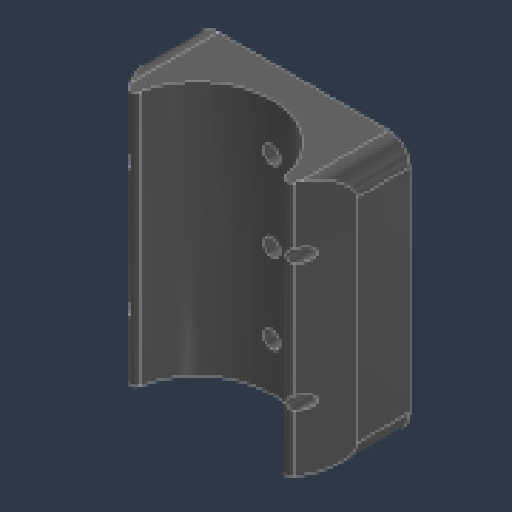
# Autodesk Inventor part: MOUNT,SPARK_MAX,ARM
Saved by Autodesk Inventor 2024.3 (Build 283343000, 343)
## iProperties
Category: _
Manager: _
ILogicPurgeVersion: 0.0.0.0
OnSaveVersion: 2.2.20.20
Created: 2025-03-14
Part Number: MOUNT,SPARK_MAX,ARM
Checked By: 00
Engr Approved By: _
User Status: Work In Process
Material: Nylon 6/6
Description: STANDARD (mm)
Document SubType Name: Modeling
Mfg Approved By: Stephen.Oerton
Designer: John Thibert
Manufacturer: Standard
Standards Organization: Custom
Density: 1.13 g/cm^3
Appearance: Dark Gray
CN_MASS: 0.0
CN_SERVICEABLE: _
FIRST_DESCRIPTION: _
SECOND_DESCRIPTION: _
THIRD_DESCRIPTION: _
ModelCat: Uncategorized
Subject: _
Author: John Thibert
Keywords: -
Revision Number: A
Autodesk Inventor part; units mm, degrees
ref_plane "YZ Plane" through (0, 0, 0) normal (1, 0, 0) x (0, 1, 0)
ref_plane "XZ Plane" through (0, 0, 0) normal (0, 1, 0) x (-1, 0, 0)
ref_plane "XY Plane" through (0, 0, 0) normal (0, 0, 1) x (1, 0, 0)
sketch "Sketch2" plane through (0, 0, 0) normal (0, 0, 1) x (1, 0, 0)
  line L0 (-31.75, -38.1) -> (31.75, -38.1)
  line L1 (31.75, -38.1) -> (31.75, 38.1)
  line L2 (31.75, 38.1) -> (-31.75, 38.1)
  line L3 (-31.75, 38.1) -> (-31.75, -38.1)
  line L4 (-31.75, -38.1) -> (31.75, 38.1) construction
  line L5 (31.75, -38.1) -> (-31.75, 38.1) construction
  point P0 (0, 0)
  dimension "d0" = 63.5
  dimension "d1" = 76.2
  constraints: 12 end point, 2 midpoint, 2 parallel, 1 horizontal, 1 perpendicular
  measures "d0" distance of L2.end L1.end
  measures "d1" distance of L0.end L1.end
extrude "Extrusion1" add sketch "Sketch2" against normal blind 31.75
sketch "Sketch4" plane through (-31.75, 38.1, 0) normal (0, 1, 0) x (1, 0, 0)
  arc A0 (53.975, 0) -> (9.525, 0) centre (31.75, 0) ccw
  line L0 (63.5, 0) -> (0, 0) construction
  line L1 (63.5, 0) -> (63.5, 31.75) projected
  line L2 (0, 31.75) -> (63.5, 31.75) projected
  line L3 (0, 0) -> (0, 31.75) projected
  line L4 (53.0485, 6.35) -> (63.5, 6.35) construction
  line L5 (0, 6.35) -> (10.4515, 6.35) construction
  line L6 (63.5, 15.875) -> (53.975, 0)
  line L7 (0, 15.875) -> (9.525, 0)
  dimension "d11" = 44.45
  dimension "d12" = 6.35
  dimension "d16" = 15.875
  constraints: 8 end point, 6 point on line, 4 point on circle, 2 midpoint, 1 centre point, 1 coincident, 1 equal length, 1 perpendicular
  measures "d11" diameter of A0
  measures "d12" distance between parallel lines of L0 L4
  measures "d16" distance from line of L2 L6.start
extrude "Extrusion2" cut sketch "Sketch4" against normal through all keep common part
fillet "Fillet1" radius 1.5875 2 edges at (-22.225, 0, 0) (22.225, 0, 0)
sketch "Sketch5" plane through (0, 0, -31.75) normal (0, 0, -1) x (-1, 0, 0)
  line L0 (25.4, 19.05) -> (-25.4, 19.05) construction
  line L1 (-25.4, 19.05) -> (-25.4, -19.05) construction
  line L2 (-25.4, -19.05) -> (25.4, -19.05) construction
  line L3 (25.4, -19.05) -> (25.4, 19.05) construction
  line L4 (25.4, 19.05) -> (-25.4, -19.05) construction
  line L5 (-25.4, 19.05) -> (25.4, -19.05) construction
  point P0 (0, 0)
  dimension "d17" = 38.1
  dimension "d18" = 50.8
  constraints: 12 end point, 2 midpoint, 2 parallel, 1 horizontal, 1 perpendicular
  measures "d17" distance of L0.end L1.end
  measures "d18" distance of L0.start L0.end
hole "Hole2" at (-25.4, 19.05, -31.75) at (25.4, -19.05, -31.75) at (25.4, 19.05, -31.75) at (-25.4, -19.05, -31.75) direction (0, 0, 1) diameter 3.9624 end through all thread size "10-32 UNF" class "2B" standard "ANSI Unified Screw Threads"
sketch "Sketch6" plane through (0, 0, -31.75) normal (0, 0, -1) x (-1, 0, 0)
  line L0 (0, -23.873) -> (0, 23.873) construction
  point P0 (0, 0)
  point P1 (0, 0)
  point P2 (0, 0)
  constraints: 4 coincident, 2 end point, 1 midpoint, 1 vertical
hole "Hole3" at (0, -23.873, -31.75) at (0, 0, -31.75) at (0, 23.873, -31.75) direction (0, 0, 1) diameter 5.1054 end through all counterbore diameter 9.525 counterbore depth 4.826 clearance for "Socket Head Cap Screw" size "#10" standard "Ansi Unified Screw Threads"
fillet "Fillet3" radius 6.35 4 edges at (-31.75, 38.1, -23.8125) (-31.75, -38.1, -23.8125) (31.75, -38.1, -23.8125) (31.75, 38.1, -23.8125)
body "Solid1"
